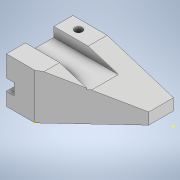
# Autodesk Inventor part: Assignment 3.3 - Angle Slider
Saved by Autodesk Inventor 2022 (Build 260153000, 153)
## iProperties
Created: 2021-05-23
Part Number: Assignment 3.3 - Angle Slider
Material: Generic
Document SubType Name: Modeling
Designer: Aaron
Density: 1 g/cm^3
Appearance: Default
Author: Aaron
Autodesk Inventor part; units mm, degrees
ref_plane "YZ Plane" through (0, 0, 0) normal (1, 0, 0) x (0, 1, 0)
ref_plane "XZ Plane" through (0, 0, 0) normal (0, 1, 0) x (-1, 0, 0)
ref_plane "XY Plane" through (0, 0, 0) normal (0, 0, 1) x (1, 0, 0)
sketch "Sketch1" plane through (0, 0, 0) normal (0, 0, 1) x (1, 0, 0)
  line L0 (0, 0) -> (-1905, 0)
  line L1 (-1905, 0) -> (-1905, 889)
  line L2 (-1905, 889) -> (-1397, 889)
  line L3 (-1397, 889) -> (-1397, 1651)
  line L4 (-1397, 1651) -> (-1905, 1651)
  line L5 (-1905, 1651) -> (-1905, 3048)
  line L6 (-1905, 3048) -> (381, 3048)
  line L7 (4826, 2413) -> (381, 3048)
  line L8 (0, 0) -> (4445, 0)
  line L9 (4445, 0) -> (4826, 0)
  line L10 (4826, 0) -> (4826, 2413)
  dimension "d0" = 1905
  dimension "d1" = 889
  dimension "d2" = 508
  dimension "d3" = 762
  dimension "d4" = 508
  dimension "d5" = 1397
  dimension "d6" = 2286
  dimension "d10" = 4445
  dimension "d11" = 381
  constraints: 22 end point, 4 perpendicular, 3 horizontal, 2 point on line, 1 vertical
  measures "d0" distance of L0.start L0.end
  measures "d1" distance of L0.end L1.end
  measures "d2" distance of L1.end L2.end
  measures "d3" distance of L2.end L3.end
  measures "d4" distance of L3.end L4.end
  measures "d5" distance of L4.end L5.end
  measures "d6" distance of L5.end L6.end
  measures "d10" distance of L0.start L8.end
  measures "d11" distance of L8.end L9.end
extrude "Extrusion1" add sketch "Sketch1" against normal blind 4445
sketch "Sketch3" plane through (-1905, 0, 0) normal (0, -1, 0) x (1, 0, 0)
  line L0 (1905, 0) -> (6731, -2786.2924)
  line L1 (6731, 0) -> (6731, -4445) projected
  line L2 (6731, -2786.2924) -> (6731, 0)
  line L3 (0, 0) -> (6731, 0) projected
  line L4 (1905, 0) -> (6731, 0)
  constraints: 6 end point, 1 collinear, 1 horizontal, 1 point on line
extrude "Extrusion2" cut sketch "Sketch3" against normal through all
sketch "Sketch4" plane through (-1905, 0, -4445) normal (0, -1, 0) x (1, 0, 0)
  point P0 (1905, 4445)
  point P1 (6731, 0)
sketch "Sketch5" plane through (0, 0, 0) normal (0, 0, 1) x (1, 0, 0)
  line L0 (381, 3048) -> (4826, 1650.986)
  line L1 (4826, 1650.986) -> (4826, 3048)
  line L2 (-1905, 3048) -> (381, 3048) projected
  line L3 (4826, 3048) -> (381, 3048)
  point P0 (0, 0)
  constraints: 6 end point, 1 perpendicular
extrude "Extrusion3" cut sketch "Sketch5" against normal through all
sketch "Sketch6" plane through (0, 0, 0) normal (0, 0, 1) x (1, 0, 0)
  line L0 (-1397, 889) -> (-1397, 1651) projected
  line L1 (4826, 1650.986) -> (4826, 0) projected
  line L2 (4826, 0) -> (0, 0) projected
  line L3 (0, 0) -> (4826, 889)
  line L4 (0, 0) -> (4826, 0)
  line L5 (4826, 889) -> (4826, 0)
  constraints: 6 end point, 1 collinear, 1 perpendicular, 1 point on line
extrude "Extrusion4" cut sketch "Sketch6" against normal through all
sketch "Sketch7" plane through (-1905, 1651, 0) normal (-1, 0, 0) x (0, 0, 1)
  line L0 (-4445, 1397) -> (-4445, -0.014) projected
  line L1 (-3175, 1397) -> (-3175, 762)
  line L2 (-3175, 762) -> (-1270, 762)
  line L3 (-1270, 762) -> (-1270, 1397)
  line L4 (-1270, 1397) -> (-3175, 1397)
  point P0 (0, -1651)
  dimension "d24" = 635
  dimension "d25" = 1905
  constraints: 8 end point, 3 perpendicular
  measures "d24" distance of L1.start L1.end
  measures "d25" distance of L1.end L2.end
extrude "Extrusion5" cut sketch "Sketch7" against normal through all
sketch "Sketch8" plane through (-1905, 3048, -4445) normal (0, 1, 0) x (1, 0, 0)
  circle A0 centre (1016, -635) radius 254
  point P0 (1905, -4445)
  dimension "d30" = 508
  constraints: 1 centre point
  measures "d30" diameter of A0
extrude "Extrusion6" cut sketch "Sketch8" against normal through all
body "Solid1"
